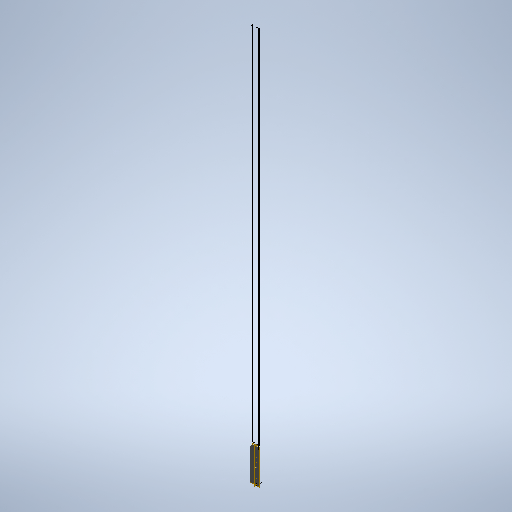
# Autodesk Inventor part: PP0735H(1)
Saved by Autodesk Inventor 2025.2 (Build 292293000, 293)
## iProperties
Category: PARTsolutions
Company: ELDON
Created: 2025-05-02
Part Number: PP0735H(1)
Material: Generic
Catalog Web Link: www.cadenas.de
Description: PP-DIN rails
Vendor: ELDON
Document SubType Name: Modeling
Designer: psAdmin
Manufacturer: ELDON
Mass: 630 g
Surface Area: 1764.71 cm^2
Volume: 84.5125 cm^3
Density: 1 g/cm^3
Appearance: PSOLRGB-175-175-175
PSOL_IDENT_0: {$CADENAS_DATA/23d-libs/eldon/common_pool/accessories/p/pp.prj},167 {VTYP=3D},{NB=PP0735H(1)},{LINA=
PSOL_IDENT_1: PP0735H},{NN=PP},{DATE=04.03.2025 09:38:01},{GEOMDATE=28.02.2025 11:58:07},{VERSION=},{LINEID=1810},
PSOL_IDENT_2: {WBVAR=DETAIL},{WBNUMERIC=DETAIL}  {NB=PP0735H(1)},{LINA=PP0735H},{KT=DUMMY},{ITEM=PP0735H},{DETAIL=
PSOL_IDENT_3: 1},{INFO=Info URL},{DES=Din rail with holes, 2000},{DES1=With holes},{MAT=Galvanized steel},{TYP=Ome
PSOL_IDENT_4: ga},{DIM=7.5 X 35},{HP=Hole pattern 18 x 5.2 mm},{MASS=0.63},{EAN=8713574013193},{TARIFFN=-},{MI=URL
PSOL_IDENT_5: },{MIALG=https://www.eldon.com/catalog-document/PP0515H/mountinginstructions/en/},{INFOPATH=https://
PSOL_IDENT_6: www.nvent.com/en-gb/catalog-document/itemsheet?pid=PP0735H},{V=1},{A=35},{A1=7.5},{A2=4.00},{A3=0.8}
PSOL_IDENT_7: ,{A4=1.8},{A5=0.00},{A6=0.0}
NB: PP0735H(1)
NN: PP
NT: DIN rails
NBSYN: $ITEM.($DETAIL.)
LINA: PP0735H
CATALOG: nVent HOFFMAN IEC-Rated Products
ITEM: PP0735H
DETAIL: high
INFO: Info URL
DES: Din rail with holes, 2000
DES1: With holes
MAT: Galvanized steel
TYP: Omega
DIM: 7.5 X 35
HP: Hole pattern 18 x 5.2 mm
MASS: 0.63
EAN: 8713574013193
MI: URL
SUPPLIER: ELDON
ARTICLENO: PP0735H(1)
BOMINFO: PP0735H
CREATOR: CADENAS GmbH
Title: PP0735H
Author: Cadenas PARTsolutions
Comments: DIN rails
Autodesk Inventor part; units mm, degrees
sketch "Sketch_2" plane through (0, 0, 0) normal (0, 1, 0) x (-1, 0, 0)
  line L0 (17.5, 6.5) -> (17.5, 7.5)
  line L1 (17.5, 7.5) -> (14.3, 7.5)
  arc A0 (14.3, 7.5) -> (12.5, 5.7) centre (14.3, 5.7) ccw
  line L2 (12.5, 5.7) -> (12.5, 1.8)
  arc A1 (11.7, 1) -> (12.5, 1.8) centre (11.7, 1.8) ccw
  line L3 (11.7, 1) -> (-11.7, 1)
  arc A2 (-12.5, 1.8) -> (-11.7, 1) centre (-11.7, 1.8) ccw
  line L4 (-12.5, 1.8) -> (-12.5, 5.7)
  arc A3 (-12.5, 5.7) -> (-14.3, 7.5) centre (-14.3, 5.7) ccw
  line L5 (-14.3, 7.5) -> (-17.5, 7.5)
  line L6 (-17.5, 7.5) -> (-17.5, 6.5)
  line L7 (-17.5, 6.5) -> (-14.3, 6.5)
  arc A4 (-13.5, 5.7) -> (-14.3, 6.5) centre (-14.3, 5.7) ccw
  line L8 (-13.5, 5.7) -> (-13.5, 1.8)
  arc A5 (-13.5, 1.8) -> (-11.7, 0) centre (-11.7, 1.8) ccw
  line L9 (-11.7, 0) -> (11.7, 0)
  arc A6 (11.7, 0) -> (13.5, 1.8) centre (11.7, 1.8) ccw
  line L10 (13.5, 1.8) -> (13.5, 5.7)
  arc A7 (14.3, 6.5) -> (13.5, 5.7) centre (14.3, 5.7) ccw
  line L11 (14.3, 6.5) -> (17.5, 6.5)
  constraints: 24 end point, 16 point on circle, 8 centre point
extrude "Extrusion1" add sketch "Sketch_2" along normal blind 160
sketch "Sketch_6" plane through (0, 0, 0) normal (0, 0, 1) x (1, 0, 0)
  arc A0 (-2.6, 6.1) -> (2.6, 6.1) centre (0, 6.1) ccw
  line L0 (2.6, 6.1) -> (2.6, 18.9)
  arc A1 (2.6, 18.9) -> (-2.6, 18.9) centre (0, 18.9) ccw
  line L1 (-2.6, 18.9) -> (-2.6, 6.1)
  constraints: 4 end point, 4 point on circle, 2 centre point
extrude "Extrusion2" cut sketch "Sketch_6" along normal blind 2
pattern_linear "Rectangular Pattern1" count 80 spacing 22.9 along (0, 1, 0) of "Extrusion2"
body "Solid1"
